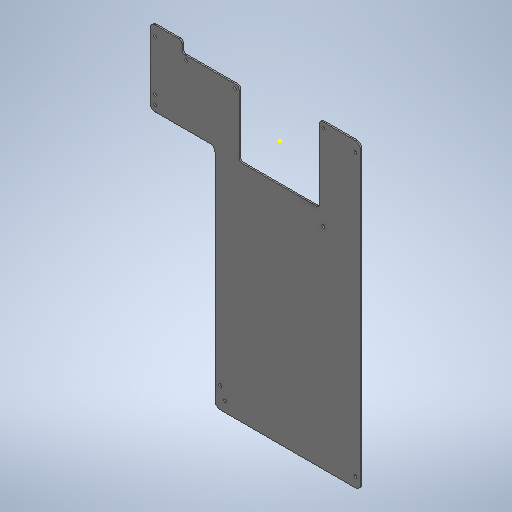
# Autodesk Inventor part: 天板
Saved by Autodesk Inventor 2026.2 (Build 302298010, 298A)
## iProperties
Created: 2026-05-07
Part Number: 天板
Material: 一般
Document SubType Name: Modeling
Designer: Yagis
Density: 1 g/cm^3
Appearance: 既定
Author: Yagis
Autodesk Inventor part; units mm, degrees
ref_plane "YZ Plane" through (0, 0, 0) normal (1, 0, 0) x (0, 1, 0)
ref_plane "XZ Plane" through (0, 0, 0) normal (0, 1, 0) x (-1, 0, 0)
ref_plane "XY Plane" through (0, 0, 0) normal (0, 0, 1) x (1, 0, 0)
sketch "スケッチ2" plane through (0, 0, 0) normal (0, 0, 1) x (1, 0, 0)
  line L0 (-75, 37.5) -> (75, 37.5)
  line L1 (80, 32.5) -> (80, -257.5)
  line L2 (75, -262.5) -> (-60, -262.5)
  line L3 (-65, -183.2657) -> (-65, -42.5)
  arc A0 (80, 32.5) -> (75, 37.5) centre (75, 32.5) ccw
  arc A1 (75, -262.5) -> (80, -257.5) centre (75, -257.5) ccw
  line L4 (-65, -257.5) -> (-65, -183.1423)
  arc A2 (-65, -257.5) -> (-60, -262.5) centre (-60, -257.5) ccw
  line L5 (-75, 37.5) -> (-125, 37.5)
  line L6 (-130, 32.5) -> (-130, -32.5)
  line L7 (-125, -37.5) -> (-70, -37.5)
  arc A3 (-125, 37.5) -> (-130, 32.5) centre (-125, 32.5) ccw
  arc A4 (-130, -32.5) -> (-125, -37.5) centre (-125, -32.5) ccw
  arc A5 (-65, -42.5) -> (-70, -37.5) centre (-70, -42.5) ccw
  point P0 (0, 0)
  point P1 (-75, 37.5)
  point P2 (80, -262.5)
  point P3 (80, 37.5)
  point P4 (-65, -262.5)
  point P5 (-75, 0)
  point P6 (0, 37.5)
  point P7 (0, 0)
  point P8 (-130, 0)
  dimension "d1" = 300
  dimension "d24" = 5
  dimension "d49" = 210
  dimension "d50" = 5
  dimension "d51" = 75
  dimension "d78" = 145
  constraints: 16 end point, 12 point on circle, 12 tangent, 8 point on line, 6 centre point, 3 perpendicular, 2 equal radius, 2 horizontal, 2 midpoint, 1 coincident, 1 collinear, 1 horizontal alignment, 1 parallel, 1 vertical, 1 vertical alignment
  measures "d1" distance of point (80, 37.5) point (80, -262.5)
  measures "d24" radius of A2
  measures "d49" distance from line of L1 point (-130, 0)
  measures "d50" radius of A3
  measures "d51" distance between parallel lines of L7 L5
  measures "d78" distance between parallel lines of L1 L4
extrude "押し出し1" add sketch "スケッチ2" along normal blind 1.5
sketch "スケッチ5" plane through (0, 0, 1.5) normal (0, 0, 1) x (1, 0, 0)
  line L0 (75, 37.5) -> (-125, 37.5) projected
  line L1 (80, -257.5) -> (80, 32.5) projected
  line L2 (-60, -262.5) -> (75, -262.5) projected
  line L3 (-130, 32.5) -> (-130, -32.5) projected
  line L4 (-125, -37.5) -> (-70, -37.5) projected
  line L5 (-65, -42.5) -> (-65, -257.5) projected
  point P0 (-125, 27.5)
  point P1 (75, 27.5)
  point P2 (75, -252.5)
  point P3 (-70, 37.5)
  point P4 (-125, -31.5)
  point P5 (-60, -241.5)
  point P6 (43, -52.5)
  point P7 (43, 32.5)
  point P8 (-45, 22.5)
  point P9 (-125, -22.5)
  point P10 (-55, -252.5)
  point P11 (-94, 22.5)
  dimension "d25" = 10
  dimension "d27" = 5
  dimension "d44" = 80
  dimension "d46" = 85
  dimension "d52" = 5
  dimension "d55" = 10
  dimension "d56" = 10
  dimension "d58" = 21
  dimension "d59" = 5
  dimension "d60" = 15
  dimension "d61" = 69
  dimension "d62" = 5
  dimension "d66" = 54
  dimension "d67" = 49
  dimension "d77" = 37
  constraints: 4 vertical alignment, 2 horizontal alignment
  measures "d25" distance from line of point (-125, 27.5) L0
  measures "d27" distance from line of L1 point (75, 27.5)
  measures "d44" horizontal distance of point (-45, 22.5) point (-125, -31.5)
  measures "d46" distance of point (43, -52.5) point (43, 32.5)
  measures "d52" distance from line of L3 point (-125, 27.5)
  measures "d55" distance from line of L2 point (-55, -252.5)
  measures "d56" distance from line of L5 point (-55, -252.5)
  measures "d58" distance from line of L2 point (-60, -241.5)
  measures "d59" distance from line of L5 point (-60, -241.5)
  measures "d60" distance from line of L4 point (-125, -22.5)
  measures "d61" distance from line of L0 point (-125, -31.5)
  measures "d62" distance from line of L0 point (43, 32.5)
  measures "d66" vertical distance of point (-45, 22.5) point (-125, -31.5)
  measures "d67" distance of point (-94, 22.5) point (-45, 22.5)
  measures "d77" distance from line of L1 point (43, 32.5)
hole "穴3" at (-125, 27.5, 1.5) at (75, 27.5, 1.5) at (75, -252.5, 1.5) at (-125, -31.5, 1.5) at (-60, -241.5, 1.5) at (-45, 22.5, 1.5) at (43, 32.5, 1.5) at (43, -52.5, 1.5) at (-125, -22.5, 1.5) at (-55, -252.5, 1.5) at (-94, 22.5, 1.5) direction (0, 0, -1) diameter 3 depth 8.1 tip angle 118
sketch "スケッチ6" plane through (0, 0, 1.5) normal (0, 0, 1) x (1, 0, 0)
  point P0 (0, 0)
sketch "スケッチ7" plane through (0, 0, 1.5) normal (0, 0, 1) x (1, 0, 0)
  line L0 (-41, 26.5) -> (-98, 26.5)
  line L1 (-98, 26.5) -> (-98, 37.5)
  line L2 (-98, 37.5) -> (39, 37.5)
  line L3 (39, 37.5) -> (39, -38.5)
  line L4 (-41, 0) -> (-41, 26.5)
  circle A0 centre (-45, 22.5) radius 1.5 projected
  circle A1 centre (-94, 22.5) radius 1.5 projected
  line L5 (75, 37.5) -> (-125, 37.5) projected
  line L6 (39, -38.5) -> (-41, -38.5)
  line L7 (-41, -38.5) -> (-41, 0)
  point P0 (-25.5, 0)
  dimension "d68" = 4
  dimension "d69" = 4
  dimension "d70" = 4
  dimension "d74" = 76
  dimension "d75" = 80
  constraints: 14 end point, 4 perpendicular, 2 horizontal, 1 collinear
  measures "d68" distance from line of L0 A0.centre
  measures "d69" distance from line of L4 A0.centre
  measures "d70" horizontal distance of L0.end A1.centre
  measures "d74" distance of L2.end L3.end
  measures "d75" distance between parallel lines of L3 L7
extrude "押し出し2" cut sketch "スケッチ7" against normal blind 10 contours L0 L1 L2 L3 L6 L7 L4
fillet "フィレット1" radius 3 6 edges at (-98, 26.5, 0.75) (-41, 26.5, 0.75) (-98, 37.5, 0.75) (-41, -38.5, 0.75) (39, -38.5, 0.75) (39, 37.5, 0.75)
